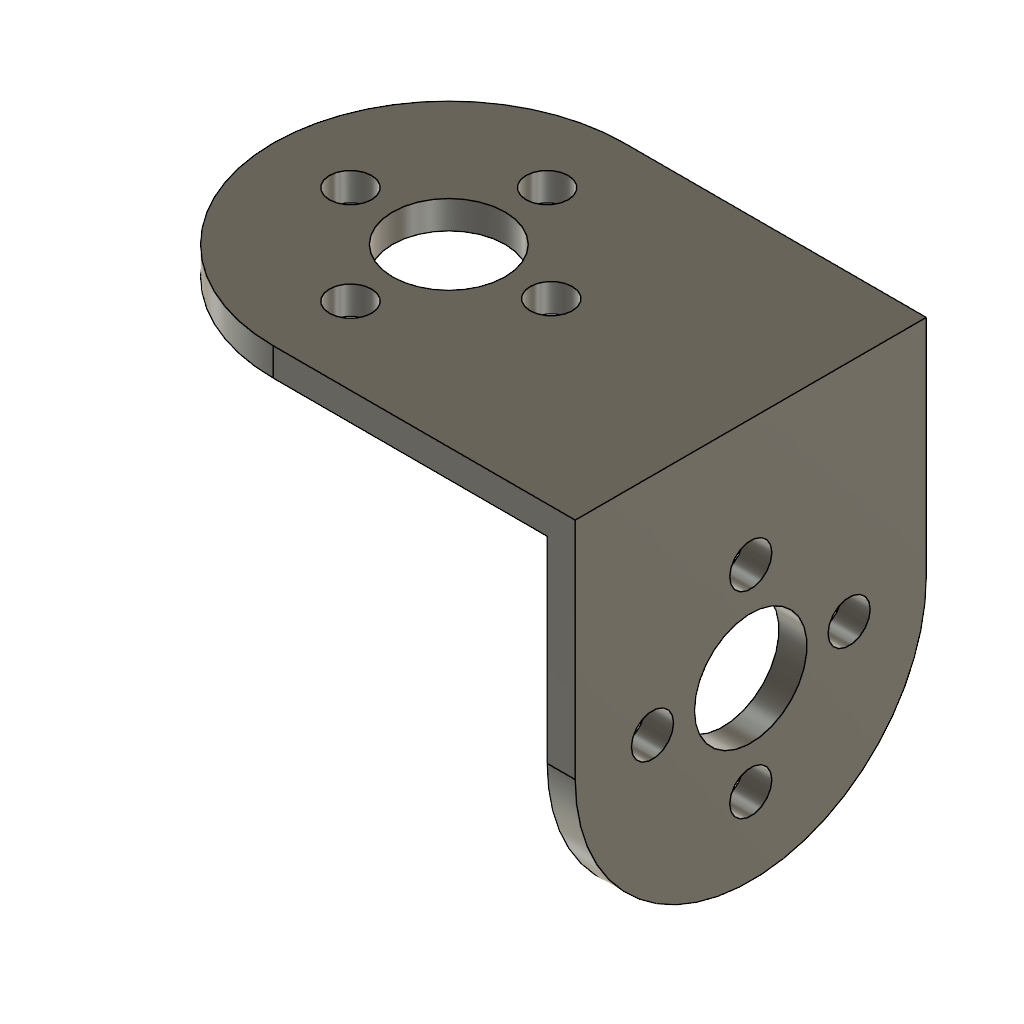
soporte_motor_12V (Autodesk Fusion 360 design; units mm, degrees)
Autodesk Fusion 360 part; units mm, degrees
sketch "Boceto1" plane through (0, 0, 0) normal (0, 0, 1) x (1, 0, 0)
  line L0 (0, 12.5) -> (0, -12.5)
  arc A0 (0, 12.5) -> (0, -12.5) centre (0, 0) ccw
  line L1 (0, 12.5) -> (19.5, 12.5)
  line L2 (0, -12.5) -> (19.5, -12.5)
  line L3 (19.5, -12.5) -> (19.5, 12.5)
  circle A1 centre (0, 0) radius 4
  circle A2 centre (0, 0) radius 7 construction
  circle A3 centre (0, 7) radius 1.5
  circle A4 centre (-7, 0) radius 1.5
  circle A5 centre (0, -7) radius 1.5
  circle A6 centre (6.9935, 0.3006) radius 1.5
  dimension "d1" = 25
  dimension "d2" = 19.5
  dimension "d3" = 19.5
  dimension "d4" = 8
  dimension "d5" = 14
  dimension "d6" = 3
  dimension "d7" = 3
  dimension "d8" = 3
  dimension "d9" = 3
  constraint coincident A0.centre A1.centre
  constraint perpendicular L0 A0
  constraint perpendicular L0 L1
  constraint perpendicular L0 L2
  constraint concentric A0 A2
  constraint coincident A2 A3.centre
  constraint coincident L0 A3.centre
  constraint coincident A2 A4.centre
  constraint coincident A2 A5.centre
  constraint coincident L0 A5.centre
  constraint coincident A2 A6.centre
  measures "d1" diameter of A0
  measures "d2" distance of L0.start L1.end
  measures "d3" distance of L0.end L2.end
  measures "d4" diameter of A1
  measures "d5" diameter of A2
  measures "d6" diameter of A3
  measures "d7" diameter of A4
  measures "d8" diameter of A5
  measures "d9" diameter of A6
extrude "Extruir1" add sketch "Boceto1" along normal blind 2 contours L0 L1 L2 L3 A1 A3 A5 | L0 A0 A1 A3 A5
sketch "Boceto2" plane through (19.5, 0, 0) normal (1, 0, 0) x (0, 1, 0)
  line L0 (-12.5, 0) -> (12.5, 0)
  line L1 (12.5, 0) -> (12.5, 2)
  line L2 (12.5, 2) -> (-12.5, 2)
  line L3 (-12.5, 2) -> (-12.5, 0)
  line L4 (12.5, 0) -> (12.5, -14)
  line L5 (-12.5, 0) -> (-12.5, -14)
  circle A0 centre (0, -14) radius 4
  circle A1 centre (0, -14) radius 7 construction
  circle A2 centre (0, -7) radius 1.5
  circle A3 centre (-7, -14) radius 1.5
  circle A4 centre (0, -21) radius 1.5
  circle A5 centre (7, -14) radius 1.5
  circle A6 centre (0, -14) radius 12.5
  line L6 (-12.5, 2) -> (12.5, 2)
  line L7 (12.5, 2) -> (12.5, 0)
  line L8 (12.5, 0) -> (-12.5, 0)
  line L9 (-12.5, 0) -> (-12.5, 2)
  dimension "d12" = 14
  dimension "d13" = 14
  dimension "d14" = 8
  dimension "d15" = 14
  dimension "d16" = 3
  dimension "d17" = 3
  dimension "d18" = 3
  dimension "d19" = 3
  constraint coincident L0.end L1.start
  constraint perpendicular L0 L4
  constraint coincident L0.start L3.end
  constraint perpendicular L0 L5
  constraint concentric A0 A1
  constraint coincident A1 A2.centre
  constraint coincident A1 A3.centre
  constraint coincident A1 A4.centre
  constraint coincident A1 A5.centre
  constraint concentric A0 A6
  constraint coincident L5.end A6
  constraint horizontal L6
  constraint vertical L7
  constraint horizontal L8
  constraint vertical L9
  constraint coincident L2.end L3.start
  measures "d12" distance of L0.end L4.end
  measures "d13" distance of L0.start L5.end
  measures "d14" diameter of A0
  measures "d15" diameter of A1
  measures "d16" diameter of A2
  measures "d17" diameter of A3
  measures "d18" diameter of A4
  measures "d19" diameter of A5
extrude "Extruir2" add sketch "Boceto2" along normal blind 2
equation "d1 = ( 12.5 * 2 ) * 1 mm"
